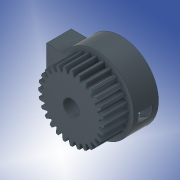
# Autodesk Inventor part: FA008
Saved by Autodesk Inventor 2017 (Build 210142000, 142)
## iProperties
Created: 2017-06-19
Part Number: FA008
Material: ABS Plastic
Document SubType Name: Modeling
Designer: Zach
Density: 1.06 g/cm^3
Appearance: CR Dark Blue
Author: Zach
Autodesk Inventor part; units mm, degrees
ref_plane "YZ Plane" through (0, 0, 0) normal (1, 0, 0) x (0, 1, 0)
ref_plane "XZ Plane" through (0, 0, 0) normal (0, 1, 0) x (-1, 0, 0)
ref_plane "XY Plane" through (0, 0, 0) normal (0, 0, 1) x (1, 0, 0)
sketch "Sketch1" plane through (0, 0, 0) normal (0, 0, 1) x (1, 0, 0)
  circle A0 centre (0, 0) radius 6.5
  circle A1 centre (0, 0) radius 22.5
  dimension "d0" = 13
  dimension "d1" = 45
  constraints: 2 centre point, 2 coincident
  measures "d0" diameter of A0
  measures "d1" diameter of A1
extrude "Extrusion1" add sketch "Sketch1" along normal blind 40
sketch "Sketch2" plane through (0, 0, 40) normal (0, 0, 1) x (1, 0, 0)
  line L0 (0, 0) -> (36.9201, 0) construction
  circle A0 centre (0, 0) radius 22.5 projected
  arc A1 (26.4109, 0.9) -> (22.4109, 2) centre (20.4718, -12.8741) ccw
  arc A2 (26.4109, -0.9) -> (26.4109, 0.9) centre (6.4312, 0) ccw
  arc A3 (22.4109, -2) -> (26.4109, -0.9) centre (20.4718, 12.8741) ccw
  arc A4 (22.4109, -2) -> (22.4109, 2) centre (0, 0) ccw
  circle A5 centre (0, 0) radius 22.5 projected
  arc A6 (25.5485, 6.7544) -> (21.404, 6.9368) centre (22.8233, -7.9959) ccw
  arc A7 (25.949, 4.9996) -> (25.5485, 6.7544) centre (6.27, 1.4311) ccw
  arc A8 (22.2941, 3.037) -> (25.949, 4.9996) centre (17.0938, 17.1068) ccw
  arc A9 (22.2941, 3.037) -> (21.404, 6.9368) centre (0, 0) ccw
  arc A10 (23.4049, 12.2701) -> (19.3238, 11.5257) centre (24.0303, -2.7168) ccw
  arc A11 (24.1859, 10.6484) -> (23.4049, 12.2701) centre (5.7943, 2.7904) ccw
  arc A12 (21.0593, 7.9218) -> (24.1859, 10.6484) centre (12.8586, 20.4816) ccw
  arc A13 (21.0593, 7.9218) -> (19.3238, 11.5257) centre (0, 0) ccw
  arc A14 (20.0878, 17.1706) -> (16.2746, 15.5367) centre (24.0324, 2.6986) ccw
  arc A15 (21.21, 15.7633) -> (20.0878, 17.1706) centre (5.0281, 4.0098) ccw
  arc A16 (18.7686, 12.4093) -> (21.21, 15.7633) centre (7.9786, 22.8294) ccw
  arc A17 (18.7686, 12.4093) -> (16.2746, 15.5367) centre (0, 0) ccw
  arc A18 (15.7633, 21.21) -> (12.4093, 18.7686) centre (22.8294, 7.9786) ccw
  arc A19 (17.1706, 20.0878) -> (15.7633, 21.21) centre (4.0098, 5.0281) ccw
  arc A20 (15.5367, 16.2746) -> (17.1706, 20.0878) centre (2.6986, 24.0324) ccw
  arc A21 (15.5367, 16.2746) -> (12.4093, 18.7686) centre (0, 0) ccw
  arc A22 (10.6484, 24.1859) -> (7.9218, 21.0593) centre (20.4816, 12.8586) ccw
  arc A23 (12.2701, 23.4049) -> (10.6484, 24.1859) centre (2.7904, 5.7943) ccw
  arc A24 (11.5257, 19.3238) -> (12.2701, 23.4049) centre (-2.7168, 24.0303) ccw
  arc A25 (11.5257, 19.3238) -> (7.9218, 21.0593) centre (0, 0) ccw
  arc A26 (4.9996, 25.949) -> (3.037, 22.2941) centre (17.1068, 17.0938) ccw
  arc A27 (6.7544, 25.5485) -> (4.9996, 25.949) centre (1.4311, 6.27) ccw
  arc A28 (6.9368, 21.404) -> (6.7544, 25.5485) centre (-7.9959, 22.8233) ccw
  arc A29 (6.9368, 21.404) -> (3.037, 22.2941) centre (0, 0) ccw
  arc A30 (-0.9, 26.4109) -> (-2, 22.4109) centre (12.8741, 20.4718) ccw
  arc A31 (0.9, 26.4109) -> (-0.9, 26.4109) centre (0, 6.4312) ccw
  arc A32 (2, 22.4109) -> (0.9, 26.4109) centre (-12.8741, 20.4718) ccw
  arc A33 (2, 22.4109) -> (-2, 22.4109) centre (0, 0) ccw
  arc A34 (-6.7544, 25.5485) -> (-6.9368, 21.404) centre (7.9959, 22.8233) ccw
  arc A35 (-4.9996, 25.949) -> (-6.7544, 25.5485) centre (-1.4311, 6.27) ccw
  arc A36 (-3.037, 22.2941) -> (-4.9996, 25.949) centre (-17.1068, 17.0938) ccw
  arc A37 (-3.037, 22.2941) -> (-6.9368, 21.404) centre (0, 0) ccw
  arc A38 (-12.2701, 23.4049) -> (-11.5257, 19.3238) centre (2.7168, 24.0303) ccw
  arc A39 (-10.6484, 24.1859) -> (-12.2701, 23.4049) centre (-2.7904, 5.7943) ccw
  arc A40 (-7.9218, 21.0593) -> (-10.6484, 24.1859) centre (-20.4816, 12.8586) ccw
  arc A41 (-7.9218, 21.0593) -> (-11.5257, 19.3238) centre (0, 0) ccw
  arc A42 (-17.1706, 20.0878) -> (-15.5367, 16.2746) centre (-2.6986, 24.0324) ccw
  arc A43 (-15.7633, 21.21) -> (-17.1706, 20.0878) centre (-4.0098, 5.0281) ccw
  arc A44 (-12.4093, 18.7686) -> (-15.7633, 21.21) centre (-22.8294, 7.9786) ccw
  arc A45 (-12.4093, 18.7686) -> (-15.5367, 16.2746) centre (0, 0) ccw
  arc A46 (-21.21, 15.7633) -> (-18.7686, 12.4093) centre (-7.9786, 22.8294) ccw
  arc A47 (-20.0878, 17.1706) -> (-21.21, 15.7633) centre (-5.0281, 4.0098) ccw
  arc A48 (-16.2746, 15.5367) -> (-20.0878, 17.1706) centre (-24.0324, 2.6986) ccw
  arc A49 (-16.2746, 15.5367) -> (-18.7686, 12.4093) centre (0, 0) ccw
  arc A50 (-24.1859, 10.6484) -> (-21.0593, 7.9218) centre (-12.8586, 20.4816) ccw
  arc A51 (-23.4049, 12.2701) -> (-24.1859, 10.6484) centre (-5.7943, 2.7904) ccw
  arc A52 (-19.3238, 11.5257) -> (-23.4049, 12.2701) centre (-24.0303, -2.7168) ccw
  arc A53 (-19.3238, 11.5257) -> (-21.0593, 7.9218) centre (0, 0) ccw
  arc A54 (-25.949, 4.9996) -> (-22.2941, 3.037) centre (-17.0938, 17.1068) ccw
  arc A55 (-25.5485, 6.7544) -> (-25.949, 4.9996) centre (-6.27, 1.4311) ccw
  arc A56 (-21.404, 6.9368) -> (-25.5485, 6.7544) centre (-22.8233, -7.9959) ccw
  arc A57 (-21.404, 6.9368) -> (-22.2941, 3.037) centre (0, 0) ccw
  arc A58 (-26.4109, -0.9) -> (-22.4109, -2) centre (-20.4718, 12.8741) ccw
  arc A59 (-26.4109, 0.9) -> (-26.4109, -0.9) centre (-6.4312, 0) ccw
  arc A60 (-22.4109, 2) -> (-26.4109, 0.9) centre (-20.4718, -12.8741) ccw
  arc A61 (-22.4109, 2) -> (-22.4109, -2) centre (0, 0) ccw
  arc A62 (-25.5485, -6.7544) -> (-21.404, -6.9368) centre (-22.8233, 7.9959) ccw
  arc A63 (-25.949, -4.9996) -> (-25.5485, -6.7544) centre (-6.27, -1.4311) ccw
  arc A64 (-22.2941, -3.037) -> (-25.949, -4.9996) centre (-17.0938, -17.1068) ccw
  arc A65 (-22.2941, -3.037) -> (-21.404, -6.9368) centre (0, 0) ccw
  arc A66 (-23.4049, -12.2701) -> (-19.3238, -11.5257) centre (-24.0303, 2.7168) ccw
  arc A67 (-24.1859, -10.6484) -> (-23.4049, -12.2701) centre (-5.7943, -2.7904) ccw
  arc A68 (-21.0593, -7.9218) -> (-24.1859, -10.6484) centre (-12.8586, -20.4816) ccw
  arc A69 (-21.0593, -7.9218) -> (-19.3238, -11.5257) centre (0, 0) ccw
  arc A70 (-20.0878, -17.1706) -> (-16.2746, -15.5367) centre (-24.0324, -2.6986) ccw
  arc A71 (-21.21, -15.7633) -> (-20.0878, -17.1706) centre (-5.0281, -4.0098) ccw
  arc A72 (-18.7686, -12.4093) -> (-21.21, -15.7633) centre (-7.9786, -22.8294) ccw
  arc A73 (-18.7686, -12.4093) -> (-16.2746, -15.5367) centre (0, 0) ccw
  arc A74 (-15.7633, -21.21) -> (-12.4093, -18.7686) centre (-22.8294, -7.9786) ccw
  arc A75 (-17.1706, -20.0878) -> (-15.7633, -21.21) centre (-4.0098, -5.0281) ccw
  arc A76 (-15.5367, -16.2746) -> (-17.1706, -20.0878) centre (-2.6986, -24.0324) ccw
  arc A77 (-15.5367, -16.2746) -> (-12.4093, -18.7686) centre (0, 0) ccw
  arc A78 (-10.6484, -24.1859) -> (-7.9218, -21.0593) centre (-20.4816, -12.8586) ccw
  arc A79 (-12.2701, -23.4049) -> (-10.6484, -24.1859) centre (-2.7904, -5.7943) ccw
  arc A80 (-11.5257, -19.3238) -> (-12.2701, -23.4049) centre (2.7168, -24.0303) ccw
  arc A81 (-11.5257, -19.3238) -> (-7.9218, -21.0593) centre (0, 0) ccw
  arc A82 (-4.9996, -25.949) -> (-3.037, -22.2941) centre (-17.1068, -17.0938) ccw
  arc A83 (-6.7544, -25.5485) -> (-4.9996, -25.949) centre (-1.4311, -6.27) ccw
  arc A84 (-6.9368, -21.404) -> (-6.7544, -25.5485) centre (7.9959, -22.8233) ccw
  arc A85 (-6.9368, -21.404) -> (-3.037, -22.2941) centre (0, 0) ccw
  arc A86 (0.9, -26.4109) -> (2, -22.4109) centre (-12.8741, -20.4718) ccw
  arc A87 (-0.9, -26.4109) -> (0.9, -26.4109) centre (0, -6.4312) ccw
  arc A88 (-2, -22.4109) -> (-0.9, -26.4109) centre (12.8741, -20.4718) ccw
  arc A89 (-2, -22.4109) -> (2, -22.4109) centre (0, 0) ccw
  arc A90 (6.7544, -25.5485) -> (6.9368, -21.404) centre (-7.9959, -22.8233) ccw
  arc A91 (4.9996, -25.949) -> (6.7544, -25.5485) centre (1.4311, -6.27) ccw
  arc A92 (3.037, -22.2941) -> (4.9996, -25.949) centre (17.1068, -17.0938) ccw
  arc A93 (3.037, -22.2941) -> (6.9368, -21.404) centre (0, 0) ccw
  arc A94 (12.2701, -23.4049) -> (11.5257, -19.3238) centre (-2.7168, -24.0303) ccw
  arc A95 (10.6484, -24.1859) -> (12.2701, -23.4049) centre (2.7904, -5.7943) ccw
  arc A96 (7.9218, -21.0593) -> (10.6484, -24.1859) centre (20.4816, -12.8586) ccw
  arc A97 (7.9218, -21.0593) -> (11.5257, -19.3238) centre (0, 0) ccw
  arc A98 (17.1706, -20.0878) -> (15.5367, -16.2746) centre (2.6986, -24.0324) ccw
  arc A99 (15.7633, -21.21) -> (17.1706, -20.0878) centre (4.0098, -5.0281) ccw
  arc A100 (12.4093, -18.7686) -> (15.7633, -21.21) centre (22.8294, -7.9786) ccw
  arc A101 (12.4093, -18.7686) -> (15.5367, -16.2746) centre (0, 0) ccw
  arc A102 (21.21, -15.7633) -> (18.7686, -12.4093) centre (7.9786, -22.8294) ccw
  arc A103 (20.0878, -17.1706) -> (21.21, -15.7633) centre (5.0281, -4.0098) ccw
  arc A104 (16.2746, -15.5367) -> (20.0878, -17.1706) centre (24.0324, -2.6986) ccw
  arc A105 (16.2746, -15.5367) -> (18.7686, -12.4093) centre (0, 0) ccw
  arc A106 (24.1859, -10.6484) -> (21.0593, -7.9218) centre (12.8586, -20.4816) ccw
  arc A107 (23.4049, -12.2701) -> (24.1859, -10.6484) centre (5.7943, -2.7904) ccw
  arc A108 (19.3238, -11.5257) -> (23.4049, -12.2701) centre (24.0303, 2.7168) ccw
  arc A109 (19.3238, -11.5257) -> (21.0593, -7.9218) centre (0, 0) ccw
  arc A110 (25.949, -4.9996) -> (22.2941, -3.037) centre (17.0938, -17.1068) ccw
  arc A111 (25.5485, -6.7544) -> (25.949, -4.9996) centre (6.27, -1.4311) ccw
  arc A112 (21.404, -6.9368) -> (25.5485, -6.7544) centre (22.8233, 7.9959) ccw
  arc A113 (21.404, -6.9368) -> (22.2941, -3.037) centre (0, 0) ccw
  circle A114 centre (0, 0) radius 7.7378
  circle A115 centre (0, 0) radius 6.5 projected
  point P0 (26.4312, 0)
  point P1 (22.5, 0)
  point P2 (25.7685, 5.8815)
  point P3 (21.9359, 5.0067)
  point P4 (23.8137, 11.4681)
  point P5 (20.2718, 9.7624)
  point P6 (20.6647, 16.4796)
  point P7 (17.5912, 14.0285)
  point P8 (16.4796, 20.6647)
  point P9 (14.0285, 17.5912)
  point P10 (11.4681, 23.8137)
  point P11 (9.7624, 20.2718)
  point P12 (5.8815, 25.7685)
  point P13 (5.0067, 21.9359)
  point P14 (0, 26.4312)
  point P15 (0, 22.5)
  point P16 (-5.8815, 25.7685)
  point P17 (-5.0067, 21.9359)
  point P18 (-11.4681, 23.8137)
  point P19 (-9.7624, 20.2718)
  point P20 (-16.4796, 20.6647)
  point P21 (-14.0285, 17.5912)
  point P22 (-20.6647, 16.4796)
  point P23 (-17.5912, 14.0285)
  point P24 (-23.8137, 11.4681)
  point P25 (-20.2718, 9.7624)
  point P26 (-25.7685, 5.8815)
  point P27 (-21.9359, 5.0067)
  point P28 (-26.4312, 0)
  point P29 (-22.5, 0)
  point P30 (-25.7685, -5.8815)
  point P31 (-21.9359, -5.0067)
  point P32 (-23.8137, -11.4681)
  point P33 (-20.2718, -9.7624)
  point P34 (-20.6647, -16.4796)
  point P35 (-17.5912, -14.0285)
  point P36 (-16.4796, -20.6647)
  point P37 (-14.0285, -17.5912)
  point P38 (-11.4681, -23.8137)
  point P39 (-9.7624, -20.2718)
  point P40 (-5.8815, -25.7685)
  point P41 (-5.0067, -21.9359)
  point P42 (0, -26.4312)
  point P43 (0, -22.5)
  point P44 (5.8815, -25.7685)
  point P45 (5.0067, -21.9359)
  point P46 (11.4681, -23.8137)
  point P47 (9.7624, -20.2718)
  point P48 (16.4796, -20.6647)
  point P49 (14.0285, -17.5912)
  point P50 (20.6647, -16.4796)
  point P51 (17.5912, -14.0285)
  point P52 (23.8137, -11.4681)
  point P53 (20.2718, -9.7624)
  point P54 (25.7685, -5.8815)
  point P55 (21.9359, -5.0067)
  dimension "d4" = 15
  dimension "d5" = 4
  dimension "d6" = 1.8
  dimension "d7" = 20
  dimension "d8" = 2
  dimension "d9" = 15
  dimension "d12" = 360
  constraints: 228 point on circle, 113 centre point, 2 end point, 2 point on line, 1 coincident, 1 concentric, 1 horizontal, 1 vertical alignment, 395 other
  measures "d4" radius of A1
  measures "d5" horizontal distance of A1.start A0.start
  measures "d6" distance of A1.start A2.start
  measures "d7" radius of A2
  measures "d8" vertical distance of point (26.431, 0) A0.start
  measures "d9" radius of A3
extrude "Extrusion3" add sketch "Sketch2" against normal blind 20 contours A0 | A0 A1 A2 A3 | A0 A6 A7 A8 | A110 A111 A112 A0 | A0 A10 A11 A12 | A106 A107 A108 A0 | A0 A14 A15 A16 | A102 A103 A104 A0 | A0 A18 A19 A20 | A98 A99 A100 A0 | A0 A22 A23 A24 | A94 A95 A96 A0 | A0 A26 A27 A28 | A90 A91 A92 A0 | A0 A30 A31 A32 | A86 A87 A88 A0 | A0 A34 A35 A36 | A82 A83 A84 A0 | A0 A38 A39 A40 | A78 A79 A80 A0 | A0 A42 A43 A44 | A74 A75 A76 A0 | A0 A46 A47 A48 | A70 A71 A72 A0 | A0 A50 A51 A52 | A66 A67 A68 A0 | A0 A54 A55 A56 | A62 A63 A64 A0 | A0 A58 A59 A60
sketch "Sketch3" plane through (0, 0, 0) normal (0, 0, -1) x (-1, 0, 0)
  line L0 (0, 15) -> (40, 15) construction
  line L1 (40, 15) -> (40, -15) construction
  line L2 (40, -15) -> (0, -15) construction
  line L3 (0, -15) -> (0, 15) construction
  line L4 (0, 15) -> (40, 15)
  line L5 (40, 15) -> (40, -15)
  line L6 (40, -15) -> (0, -15)
  line L7 (0, -15) -> (0, -6.5)
  circle A0 centre (0, 0) radius 6.5 projected
  line L8 (0, 15) -> (0, 6.5)
  arc A1 (0, -6.5) -> (0, 6.5) centre (0, 0) ccw
  dimension "d18" = 40
  dimension "d19" = 30
  constraints: 18 end point, 5 equal length, 4 point on circle, 2 concentric, 2 point on line, 1 centre point, 1 coincident, 1 horizontal, 1 midpoint, 1 perpendicular
  measures "d18" distance of L1.end L2.end
  measures "d19" distance of L0.end L1.end
extrude "Extrusion4" add sketch "Sketch3" against normal blind 20 contours L4 L5 L6 L7 A0 L8
sketch "Sketch4" plane through (0, 0, 0) normal (0, 0, -1) x (-1, 0, 0)
  circle A0 centre (0, 0) radius 30
  circle A1 centre (0, 0) radius 6.5 projected
  dimension "d22" = 60
  constraints: 1 centre point, 1 coincident
  measures "d22" diameter of A0
extrude "Extrusion5" add sketch "Sketch4" against normal blind 20
sketch "Sketch5" plane through (-40, -15, 0) normal (-1, 0, 0) x (0, 0, 1)
  line L0 (0, 30) -> (20, 30) projected
  circle A0 centre (10, 27.7) radius 1
  circle A1 centre (10, 2.3) radius 1
  line L1 (10, 27.7) -> (10, 2.3) construction
  line L2 (20, 30) -> (20, 0) construction
  line L3 (16, 26) -> (4, 26)
  line L4 (4, 26) -> (4, 4)
  line L5 (4, 4) -> (16, 4)
  line L6 (16, 4) -> (16, 26)
  point P0 (0, 15)
  point P1 (10, 30)
  point P2 (10, 30)
  point P3 (20, 15)
  point P4 (10, 15)
  point P5 (10, 30)
  point P6 (16, 15)
  point P7 (10, 26)
  point P8 (10, 30)
  dimension "d25" = 2
  dimension "d26" = 2
  dimension "d27" = 25.4
  dimension "d28" = 22
  dimension "d29" = 12
  constraints: 10 end point, 8 midpoint, 2 centre point, 2 horizontal alignment, 2 parallel, 2 vertical alignment, 1 coincident, 1 horizontal, 1 perpendicular, 1 vertical
  measures "d25" diameter of A0
  measures "d26" diameter of A1
  measures "d27" distance of L1.end L1.start
  measures "d28" distance of L5.end L3.start
  measures "d29" distance between parallel lines of L4 L6
extrude "Extrusion6" cut sketch "Sketch5" against normal blind 20
sketch "Sketch6" plane through (-40, -11, 16) normal (0, 0, -1) x (-1, 0, 0)
  line L0 (0, 22) -> (0, 0) projected
  line L1 (0, 22) -> (-20, 22) projected
  line L2 (-20, 22) -> (-20, 0) projected
  line L3 (0, 0) -> (-20, 0) projected
  line L4 (-20, 5) -> (-15, 0)
  line L5 (-40, 11) -> (-40, -49) construction
  line L6 (-40, 11) -> (20, 11) construction
  line L7 (-20, 5) -> (-40, -6.547)
  line L8 (-20, 5) -> (3.094, 5) construction
  line L9 (-15, 0) -> (-40, -14.4338)
  line L10 (-15, 0) -> (13.8675, 0) construction
  line L11 (-40, -6.547) -> (-69.9991, 10.773)
  line L12 (-40, -14.4338) -> (-68.6521, 2.1085)
  arc A0 (-69.9991, 10.773) -> (-68.6521, 2.1085) centre (-40, 11) ccw
  arc A1 (-14.0192, 26) -> (-14.0192, -4) centre (-40, 11) ccw construction
  dimension "d32" = 5
  dimension "d33" = 45
  dimension "d34" = 60
  dimension "d35" = 90
  dimension "d36" = 150
  dimension "d37" = 150
  dimension "d38" = 120
  constraints: 18 end point, 4 point on line, 3 equal length, 3 horizontal, 2 point on circle, 1 centre point, 1 parallel, 1 vertical
  measures "d32" distance of L2.end L4.start
  measures "d33" angle of L4 L2
  measures "d34" distance of L5.start L5.end
  measures "d35" angle of L5 L6
  measures "d36" angle of L7 L8
  measures "d37" angle of L9 L10
  measures "d38" angle of L5 L12
extrude "Extrusion7" cut sketch "Sketch6" along normal through all contours L9 L12 A0 L11 L7 L2 L3 | L3 L2 L4
sketch "Sketch8" plane through (0, 0, 0) normal (0, 0, -1) x (-1, 0, 0)
  arc A0 (25.9808, 15) -> (-29.9991, -0.227) centre (0, 0) ccw projected
  line L0 (-29.9991, -0.227) -> (0, -17.547) projected
  line L1 (0, -17.547) -> (20, -6) projected
  line L2 (20, -6) -> (25, -11) projected
  line L3 (25, -11) -> (0, -25.4338) projected
  line L4 (0, -25.4338) -> (-28.6521, -8.8915) projected
  arc A1 (-28.6521, -8.8915) -> (25.9808, -15) centre (0, 0) ccw projected
  line L5 (25.9808, -15) -> (40, -15) projected
  line L6 (40, -15) -> (40, 15) projected
  line L7 (40, 15) -> (25.9808, 15) projected
  arc A2 (25.9808, 15) -> (-29.9991, -0.227) centre (0, 0) ccw projected
  circle A3 centre (0, 0) radius 6.5 projected
  arc A4 (-29.9991, -0.227) -> (-28.6521, -8.8915) centre (0, 0) ccw
  constraints: 2 point on circle, 1 centre point
extrude "Extrusion8" add sketch "Sketch8" against normal blind 5 contours L0 L1 L2 L3 L4 A4
sketch "Sketch9" plane through (0, 0, 0) normal (0, 0, -1) x (-1, 0, 0)
  line L0 (-28.6521, -8.8915) -> (0, -25.4338) projected
  line L1 (0, -17.547) -> (-29.9991, -0.227) projected
  line L2 (20, -6) -> (0, -17.547) projected
  line L3 (0, -25.4338) -> (25, -11) projected
  line L4 (40, -11) -> (25, -11) projected
  line L5 (20, -6) -> (20, 11) projected
  line L6 (40, 11) -> (20, 11) projected
  line L7 (-20, -6) -> (-20, -13.8868)
  line L8 (-8, -20.815) -> (-8, -12.9282)
  point P0 (0, 0)
  dimension "d43" = 12
  constraints: 4 end point, 4 point on line, 1 horizontal alignment, 1 parallel, 1 vertical
  measures "d43" distance between parallel lines of L8 L7
extrude "Extrusion9" cut sketch "Sketch9" against normal blind 10
body "Solid1"
